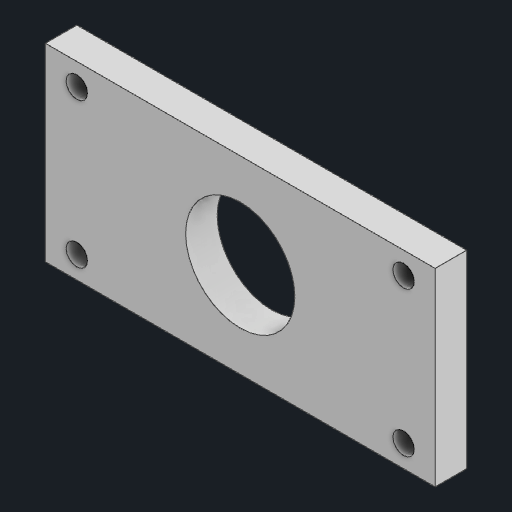
# Autodesk Inventor part: CenterPointBracket
Saved by Autodesk Inventor 2023 (Build 270158000, 158)
## iProperties
Created: 2022-12-08
Part Number: CenterPointBracket
Material: Generic
Document SubType Name: Modeling
Designer: Izack Waczko
Density: 1 g/cm^3
Appearance: Default
Author: Izack Waczko
Autodesk Inventor part; units mm, degrees
ref_plane "YZ Plane" through (0, 0, 0) normal (1, 0, 0) x (0, 1, 0)
ref_plane "XZ Plane" through (0, 0, 0) normal (0, 1, 0) x (-1, 0, 0)
ref_plane "XY Plane" through (0, 0, 0) normal (0, 0, 1) x (1, 0, 0)
sketch "Sketch1" plane through (0, 0, 0) normal (0, 0, 1) x (1, 0, 0)
  circle A0 centre (0, -32.5) radius 1.7 projected
  circle A1 centre (0, 11.5) radius 1.7 projected
  circle A2 centre (0, -11.5) radius 1.7 projected
  line L0 (5, 15) -> (-5, 15) projected
  line L1 (-5, 15) -> (-5, -15) projected
  line L2 (-5, -15) -> (5, -15) projected
  line L3 (5, -15) -> (5, 15) projected
  circle A3 centre (-51.8, 11.5) radius 1.7 projected
  circle A4 centre (-51.8, -11.5) radius 1.7 projected
  line L4 (-46.8, 15) -> (-56.8, 15) projected
  line L5 (-56.8, 15) -> (-56.8, -15) projected
  line L6 (-56.8, -15) -> (-46.8, -15) projected
  line L7 (-46.8, -15) -> (-46.8, 15) projected
  line L8 (-56.8, 15) -> (5, 15)
  line L9 (5, 15) -> (5, -15)
  line L10 (5, -15) -> (-56.8, -15)
  line L11 (-56.8, -15) -> (-56.8, 15)
  line L12 (-5, 0) -> (-46.8, 0) construction
  line L13 (-25.9, -15) -> (-25.9, 15) construction
  circle A5 centre (-25.9, 0) radius 8.65
  point P0 (0, 0)
  point P1 (-5, 15)
  point P2 (-46.8, 15)
  point P3 (-46.8, -15)
  point P4 (-5, -15)
  point P5 (-46.8, -15)
  point P6 (-56.8, -15)
  point P7 (-5, 15)
  point P8 (-46.8, 15)
  point P9 (-56.8, -15)
  dimension "d0" = 17.3
  constraints: 12 end point, 5 midpoint, 2 parallel, 1 centre point, 1 horizontal, 1 perpendicular
  measures "d0" diameter of A5
extrude "Extrusion1" add sketch "Sketch1" along normal blind 5 contours L3 L2 L1 L0 | L1 L10 L7 L8 | L7 L6 L5 L4
body "Solid1"
